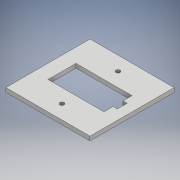
# Autodesk Inventor part: Servo Holder BOTTOM
Saved by Autodesk Inventor 2017 (Build 210142000, 142)
## iProperties
Created: 2021-03-08
Part Number: Servo Holder BOTTOM
Material: Generic
Document SubType Name: Modeling
Designer: Lenovo Y900
Density: 1 g/cm^3
Appearance: Default
Author: Lenovo Y900
Autodesk Inventor part; units mm, degrees
ref_plane "YZ Plane" through (0, 0, 0) normal (1, 0, 0) x (0, 1, 0)
ref_plane "XZ Plane" through (0, 0, 0) normal (0, 1, 0) x (-1, 0, 0)
ref_plane "XY Plane" through (0, 0, 0) normal (0, 0, 1) x (1, 0, 0)
sketch "Sketch1" plane through (0, 0, 0) normal (0, 0, 1) x (1, 0, 0)
  line L0 (-20, 10) -> (20, 10)
  line L1 (20, -10) -> (-20, -10)
  line L2 (-20, -10) -> (-20, 10)
  line L3 (-20, 10) -> (20, -10) construction
  line L4 (20, 10) -> (-20, -10) construction
  line L5 (-30, -30) -> (30, -30)
  line L6 (30, -30) -> (30, 30)
  line L7 (30, 30) -> (-30, 30)
  line L8 (-30, 30) -> (-30, -30)
  line L9 (-30, -30) -> (30, 30) construction
  line L10 (30, -30) -> (-30, 30) construction
  line L11 (0, 10) -> (0, 20)
  line L12 (0, -10) -> (0, -20)
  circle A0 centre (0, 20) radius 1.5
  circle A1 centre (0, -20) radius 1.5
  line L13 (20, -3.5) -> (23, -3.5)
  line L14 (23, -3.5) -> (23, 3.5)
  line L15 (23, 3.5) -> (20, 3.5)
  line L16 (20, 10) -> (20, 3.5)
  line L17 (20, -3.5) -> (20, -10)
  point P0 (0, 0)
  point P1 (20, 0)
  dimension "d0" = 40
  dimension "d1" = 20
  dimension "d2" = 60
  dimension "d3" = 60
  dimension "d4" = 10
  dimension "d5" = 10
  dimension "d6" = 3
  dimension "d7" = 3
  dimension "d11" = 7
  constraints: 36 end point, 6 midpoint, 6 parallel, 4 perpendicular, 3 horizontal, 2 centre point, 2 coincident, 2 vertical
  measures "d0" distance of L1.start L1.end
  measures "d1" distance of L0.end L1.start
  measures "d2" distance of L7.end L6.end
  measures "d3" distance of L6.end L5.end
  measures "d4" distance of L11.start L11.end
  measures "d5" distance of L12.start L12.end
  measures "d6" diameter of A0
  measures "d7" diameter of A1
  measures "d11" distance of L14.end L13.end
extrude "Extrusion2" add sketch "Sketch1" along normal blind 3
body "Solid2"
